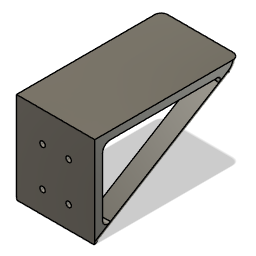
xAxisMotorMount v2 (Autodesk Fusion 360 archive; units mm, degrees)
design "xAxisMotorMount" references "MOTOR STEPER NEMA 23"
Autodesk Fusion 360 part; units mm, degrees
sketch "Sketch1" plane through (0, 0, 0) normal (1, 0, 0) x (0, 0, -1)
  line L0 (0, 28.2) -> (111, 28.2)
  line L1 (111, 28.2) -> (111, -28.2)
  line L2 (111, -28.2) -> (0, -28.2)
  line L3 (0, -28.2) -> (0, 28.2)
  line L4 (0, -28.2) -> (0, -98.2)
  line L5 (0, -98.2) -> (6, -98.2)
  line L6 (0, -28.2) -> (0, -34.2)
  line L7 (6, -34.2) -> (111, -34.2)
  line L8 (111, -28.2) -> (111, -34.2)
  line L9 (6, -92.3444) -> (6, -34.2)
  line L10 (6, -98.2) -> (111, -34.2)
  line L11 (6, -92.3444) -> (6, -90)
  line L12 (6, -92.3444) -> (101.3932, -34.2)
  line L13 (6, -92.3444) -> (6, -98.2)
  dimension "d1" = 70
  dimension "d2" = 6
  dimension "d3" = 6
  dimension "d4" = 6
  constraint horizontal L0
  constraint vertical L1
  constraint horizontal L2
  constraint vertical L3
  constraint perpendicular L2 L4
  constraint perpendicular L4 L5
  constraint coincident L4 L6.end
  constraint perpendicular L1 L7
  constraint perpendicular L7 L8
  constraint perpendicular L7 L9
  constraint coincident L9 L11.end
  constraint coincident L7 L12.end
  constraint perpendicular L5 L13
  measures "d1" distance of L2.end L4.end
  measures "d2" distance of L2.end L6.end
  measures "d3" distance of L4.end L5.end
  measures "d4" distance of L1.end L7.end
extrude "Extrude1" add sketch "Sketch1" along normal mid plane 60 contours L2 L4 L5 L6 L7 L8 L9 L11 L13 | L7 L10 L12 L13
sketch "Sketch2" plane through (0, -74.2659, -45.2668) normal (0, -0.853884, -0.520463) x (-1, 0, 0)
  line L0 (30, 76.9813) -> (-30, 76.9813)
  line L1 (-30, 76.9813) -> (-30, -45.9861)
  line L2 (-30, -45.9861) -> (30, -45.9861)
  line L3 (30, -45.9861) -> (30, 76.9813)
  line L4 (-16, 62.9813) -> (-16, -31.9861)
  line L5 (-16, -31.9861) -> (16, -31.9861)
  line L6 (16, -31.9861) -> (16, 62.9813)
  line L7 (16, 62.9813) -> (-16, 62.9813)
  dimension "d10" = -14
extrude "Extrude2" cut sketch "Sketch2" against normal up to surface (5 mm away) contours L4 L5 L6 L7
sketch "Sketch3" plane through (0, 0, -6) normal (0, 0, -1) x (-1, 0, 0)
  line L0 (30, -34.2) -> (-30, -34.2)
  line L1 (-30, -34.2) -> (-30, -92.3444)
  line L2 (-30, -92.3444) -> (30, -92.3444)
  line L3 (30, -92.3444) -> (30, -34.2)
  line L4 (16, -41.4865) -> (16, -90.9135)
  line L5 (16, -90.9135) -> (-16, -90.9135)
  line L6 (-16, -90.9135) -> (-16, -41.4865)
  line L7 (-16, -41.4865) -> (16, -41.4865)
  line L8 (30, -34.2) -> (-30, -34.2)
  line L9 (-30, -34.2) -> (-30, -98.2)
  line L10 (-30, -98.2) -> (30, -98.2)
  line L11 (30, -98.2) -> (30, -34.2)
  line L12 (-16, -41.4865) -> (16, -90.9135) construction
  line L13 (-10, -51.2) -> (10, -51.2) construction
  line L14 (10, -51.2) -> (10, -81.2) construction
  line L15 (10, -81.2) -> (-10, -81.2) construction
  line L16 (-10, -81.2) -> (-10, -51.2) construction
  line L17 (-10, -51.2) -> (10, -81.2) construction
  line L18 (10, -51.2) -> (-10, -81.2) construction
  circle A0 centre (-10, -51.2) radius 2.1
  circle A1 centre (10, -51.2) radius 2.1
  circle A2 centre (-10, -81.2) radius 2.1
  circle A3 centre (10, -81.2) radius 2.1
  point P0 (0, -66.2)
  dimension "d13" = 20
  dimension "d14" = 30
  dimension "d15" = 4.2
  dimension "d16" = 4.2
  dimension "d17" = 4.2
  dimension "d18" = 4.2
  constraint coincident L6.end L7.start
  constraint coincident L4.end L5.start
  constraint horizontal L13
  constraint perpendicular L13 L14
  constraint parallel L13 L15
  constraint parallel L14 L16
  constraint coincident L17 P0
  constraint coincident L18 P0
  constraint midpoint L12 P0
  constraint coincident L13.start L16.end
  constraint coincident L13.end L14.start
  constraint coincident L15.end L16.start
  constraint coincident L14.end L15.start
  measures "d13" distance of L14.end L15.end
  measures "d14" distance of L13.end L14.end
  measures "d15" diameter of A0
  measures "d16" diameter of A1
  measures "d17" diameter of A2
  measures "d18" diameter of A3
extrude "Extrude3" cut sketch "Sketch3" against normal blind 15 contours A0 | A1 | A2 | A3
fillet "Fillet1" radius 12.5 1 edges at (0, -34.2, -111)
fillet "Fillet2" radius 5 4 edges at (30, -68.0134, -55.5248) (30, -33.7254, -109.1767) (-30, -33.7254, -109.1767) (-30, -68.0134, -55.5248)
fillet "Fillet3" radius 6 1 edges at (0, -34.2, -6)
fillet "Fillet4" radius 2 1 edges at (0, -34.2, -101.3932)
fillet "Fillet5" radius 4 1 edges at (0, -92.3444, -6)
